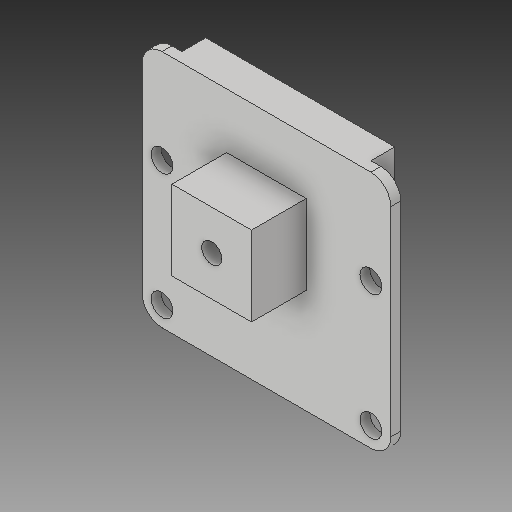
# Autodesk Inventor part: RaspberryPiCameraModel
Saved by Autodesk Inventor 2019.3 (Build 233278000, 278)
## iProperties
Created: 2018-12-24
Part Number: RaspberryPiCameraModel
Material: Generic
Document SubType Name: Modeling
Designer: steele
Density: 1 g/cm^3
Appearance: Default
Author: steele
Autodesk Inventor part; units mm, degrees
ref_plane "YZ Plane" through (0, 0, 0) normal (1, 0, 0) x (0, 1, 0)
ref_plane "XZ Plane" through (0, 0, 0) normal (0, 1, 0) x (-1, 0, 0)
ref_plane "XY Plane" through (0, 0, 0) normal (0, 0, 1) x (1, 0, 0)
sketch "Sketch1" plane through (0, 0, 0) normal (0, 0, 1) x (1, 0, 0)
  line L0 (-12.5, -12.021) -> (12.5, -12.021)
  line L1 (12.5, -12.021) -> (12.5, 12.021)
  line L2 (12.5, 12.021) -> (-12.5, 12.021)
  line L3 (-12.5, 12.021) -> (-12.5, -12.021)
  line L4 (-12.5, -12.021) -> (12.5, 12.021) construction
  line L5 (12.5, -12.021) -> (-12.5, 12.021) construction
  line L6 (-10.5, -10.021) -> (10.5, -10.021) construction
  line L7 (10.5, -10.021) -> (10.5, 2.559) construction
  line L8 (10.5, 2.559) -> (-10.5, 2.559) construction
  line L9 (-10.5, 2.559) -> (-10.5, -10.021) construction
  circle A0 centre (-10.5, -10.021) radius 1.1
  circle A1 centre (-10.5, 2.559) radius 1.1
  circle A2 centre (10.5, 2.559) radius 1.1
  circle A3 centre (10.5, -10.021) radius 1.1
  point P0 (0, 0)
  dimension "d0" = 2
  dimension "d1" = 2
  dimension "d2" = 2
  dimension "d3" = 12.58
  dimension "d4" = 9.462
  dimension "d5" = 25
  dimension "d6" = 2.2
  constraints: 20 end point, 4 centre point, 4 coincident, 4 parallel, 3 equal radius, 2 horizontal, 2 midpoint, 2 perpendicular
  measures "d0" distance between parallel lines of L6 L0
  measures "d1" distance between parallel lines of L3 L9
  measures "d2" distance between parallel lines of L7 L1
  measures "d3" distance between parallel lines of L8 L6
  measures "d4" distance between parallel lines of L2 L8
  measures "d5" distance between parallel lines of L1 L3
  measures "d6" diameter of A1
extrude "Extrusion1" add sketch "Sketch1" against normal blind 1
sketch "Sketch2" plane through (0, 0, 0) normal (0, 0, 1) x (1, 0, 0)
  line L0 (-4, -1.521) -> (4, -1.521)
  line L1 (4, -1.521) -> (4, 6.479)
  line L2 (4, 6.479) -> (-4, 6.479)
  line L3 (-4, 6.479) -> (-4, -1.521)
  line L4 (-4, -1.521) -> (4, 6.479) construction
  line L5 (4, -1.521) -> (-4, 6.479) construction
  line L6 (-12.5, -12.021) -> (12.5, -12.021) projected
  point P0 (0, 0)
  point P1 (0, 2.479)
  dimension "d9" = 14.5
  dimension "d10" = 8
  constraints: 12 end point, 2 midpoint, 2 parallel, 2 perpendicular, 1 horizontal
  measures "d9" distance from line of point (0, 2.479) L6
  measures "d10" distance of L2.end L0.start
extrude "Extrusion2" add sketch "Sketch2" along normal blind 5.5
sketch "Sketch5" plane through (0, 0, 5.5) normal (0, 0, 1) x (1, 0, 0)
  line L0 (-4, -1.521) -> (-4, 6.479) construction
  line L1 (-4, -1.521) -> (4, -1.521) construction
  line L2 (-4, 6.479) -> (4, -1.521) construction
  line L3 (4, 6.479) -> (-4, 6.479) construction
  line L4 (4, 6.479) -> (-4, -1.521) construction
  circle A0 centre (0, 2.479) radius 1
  line L5 (0, 6.479) -> (0, -1.521) construction
  point P0 (0, 0)
  dimension "d13" = 2
  constraints: 6 end point, 3 midpoint, 1 centre point
  measures "d13" diameter of A0
extrude "Extrusion3" cut sketch "Sketch5" against normal through all
fillet "Fillet1" radius 2 4 edges at (-12.5, 12.021, -0.5) (12.5, 12.021, -0.5) (12.5, -12.021, -0.5) (-12.5, -12.021, -0.5)
sketch "Sketch6" plane through (0, 0, -1) normal (0, 0, -1) x (-1, 0, 0)
  line L0 (10.5, 12.021) -> (-10.5, 12.021) construction
  line L1 (0, 12.021) -> (0, -12.021) construction
  line L2 (-10.5, -12.021) -> (10.5, -12.021) construction
  line L3 (-9.5, 7.021) -> (9.5, 7.021)
  line L4 (9.5, 7.021) -> (9.5, 12.021)
  line L5 (9.5, 12.021) -> (-9.5, 12.021)
  line L6 (-9.5, 12.021) -> (-9.5, 7.021)
  line L7 (-9.5, 7.021) -> (9.5, 12.021) construction
  line L8 (9.5, 7.021) -> (-9.5, 12.021) construction
  point P0 (0, 0)
  point P1 (0, 9.521)
  dimension "d17" = 5
  dimension "d18" = 19
  constraints: 14 end point, 4 midpoint, 2 parallel, 2 perpendicular, 1 collinear, 1 point on line
  measures "d17" distance of L5.end L3.start
  measures "d18" distance between parallel lines of L4 L6
extrude "Extrusion4" add sketch "Sketch6" along normal blind 2.4
body "Solid1"
